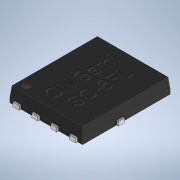
# Autodesk Inventor part: SO-8FL
Saved by Autodesk Inventor 2020.1 (Build 241239000, 239)
## iProperties
Created: 2020-03-12
Part Number: SO-8FL
Material: Generic
Document SubType Name: Modeling
Designer: yusaku
Density: 1 g/cm^3
Appearance: Default
Author: yusaku
Autodesk Inventor part; units mm, degrees
ref_plane "YZ Plane" through (0, 0, 0) normal (1, 0, 0) x (0, 1, 0)
ref_plane "XZ Plane" through (0, 0, 0) normal (0, 1, 0) x (-1, 0, 0)
ref_plane "Work Plane1" through (0, 0, 1) normal (0, 0, 1) x (1, 0, 0)
sketch "Sketch1" plane through (0, 0, 1) normal (0, 0, 1) x (1, 0, 0)
  line L0 (-2.45, 2.95) -> (2.45, 2.95)
  line L1 (2.45, 2.95) -> (2.45, -2.95)
  line L2 (2.45, -2.95) -> (-2.45, -2.95)
  line L3 (-2.45, -2.95) -> (-2.45, 2.95)
  point P0 (0, 0)
  point P1 (2.45, 0)
  point P2 (0, 2.95)
  dimension "d2" = 4.9
  dimension "d3" = 5.9
  constraints: 8 end point, 2 midpoint, 2 parallel, 1 horizontal, 1 horizontal alignment, 1 perpendicular, 1 vertical alignment
  measures "d2" distance of L0.start L0.end
  measures "d3" distance of L0.end L1.end
extrude "Extrusion1" add sketch "Sketch1" against normal blind 0.99
sketch "Sketch2" plane through (0, 0, 0) normal (0, 0, 1) x (1, 0, 0)
  line L0 (2.11, -2.5) -> (1.7, -2.5)
  line L1 (1.7, -2.5) -> (1.7, -3.075)
  line L2 (1.7, -3.075) -> (2.11, -3.075)
  line L3 (2.11, -3.075) -> (2.11, -2.5)
  line L4 (0.84, -2.5) -> (0.43, -2.5)
  line L5 (0.43, -2.5) -> (0.43, -3.075)
  line L6 (0.43, -3.075) -> (0.84, -3.075)
  line L7 (0.84, -3.075) -> (0.84, -2.5)
  line L8 (-0.43, -2.5) -> (-0.84, -2.5)
  line L9 (-0.84, -2.5) -> (-0.84, -3.075)
  line L10 (-0.84, -3.075) -> (-0.43, -3.075)
  line L11 (-0.43, -3.075) -> (-0.43, -2.5)
  line L12 (-1.7, -2.5) -> (-2.11, -2.5)
  line L13 (-2.11, -2.5) -> (-2.11, -3.075)
  line L14 (-2.11, -3.075) -> (-1.7, -3.075)
  line L15 (-1.7, -3.075) -> (-1.7, -2.5)
  line L16 (2.11, 3.075) -> (2.11, 2.075)
  line L17 (2.11, 2.075) -> (2, 2.075)
  line L18 (2, 2.075) -> (2, -0.245)
  line L19 (2, -0.245) -> (2.575, -0.245)
  line L20 (2.575, -0.245) -> (2.575, -0.655)
  line L21 (2.575, -0.655) -> (2, -0.655)
  line L22 (2, -0.655) -> (2, -1.15)
  line L23 (2, -1.15) -> (-2, -1.15)
  line L24 (-2, -1.15) -> (-2, -0.655)
  line L25 (-2, -0.655) -> (-2.575, -0.655)
  line L26 (-2.575, -0.655) -> (-2.575, -0.245)
  line L27 (-2.575, -0.245) -> (-2, -0.245)
  line L28 (-2, -0.245) -> (-2, 2.075)
  line L29 (-2.11, 2.075) -> (-2, 2.075)
  line L30 (-2.11, 2.075) -> (-2.11, 3.075)
  line L31 (2.11, 3.075) -> (1.7, 3.075)
  line L32 (1.7, 3.075) -> (1.7, 2.5)
  line L33 (1.7, 2.5) -> (-1.7, 2.5)
  line L34 (-1.7, 2.5) -> (-1.7, 3.075)
  line L35 (-1.7, 3.075) -> (-2.11, 3.075)
  line L36 (-0.635, -2.5) -> (-0.635, -3.075) construction
  line L37 (-1.905, -2.5) -> (-1.905, -3.075) construction
  line L38 (0.635, -2.5) -> (0.635, -3.075) construction
  line L39 (1.905, -2.5) -> (1.905, -3.075) construction
  line L40 (-2.45, 2.95) -> (2.45, 2.95) construction
  line L41 (0, 2.95) -> (0, -2.95) construction
  line L42 (2.45, -2.95) -> (-2.45, -2.95) construction
  line L43 (2.575, -0.45) -> (-2.575, -0.45) construction
  line L44 (-2.11, 2.075) -> (-2.11, -2.5) construction
  point P0 (0, 0)
  point P1 (0, -1.15)
  point P2 (0, 2.5)
  dimension "d6" = 0.635
  dimension "d7" = 1.27
  dimension "d10" = 1.27
  dimension "d11" = 1.35
  dimension "d12" = 0.575
  dimension "d13" = 6.15
  dimension "d14" = 5.15
  dimension "d15" = 0.125
  dimension "d16" = 3.4
  dimension "d17" = 4
  dimension "d18" = 0.41
  dimension "d19" = 0.575
  dimension "d20" = 1
  constraints: 86 end point, 19 point on line, 17 perpendicular, 14 midpoint, 8 parallel, 7 equal length, 5 horizontal, 3 vertical, 1 other
  measures "d6" distance from line of L36 point (0, 0)
  measures "d7" distance between parallel lines of L38 L36
  measures "d10" distance between parallel lines of L38 L39
  measures "d11" distance between parallel lines of L12 L23
  measures "d12" distance of L12.end L13.end
  measures "d13" distance between parallel lines of L2 L31
  measures "d14" distance between parallel lines of L26 L20
  measures "d15" distance between parallel lines of L40 L35
  measures "d16" distance between parallel lines of L40 L43
  measures "d17" distance between parallel lines of L18 L28
  measures "d18" distance of L13.end L14.end
  measures "d19" distance between parallel lines of L33 L31
  measures "d20" distance of L29.start L30.end
extrude "Extrusion2" add sketch "Sketch2" along normal blind 0.28
chamfer "Chamfer1" distance 0.0757 angle 84 4 edges at (0, 2.95, 1) (2.45, 0, 1) (0, -2.95, 1) (-2.45, 0, 1) measured on face at (0, -2.45, 1) measured on face at (1.95, 0, 1) measured on face at (0, 2.45, 1) measured on face at (-1.95, 0, 1)
sketch "Sketch3" plane through (0, 0, 1) normal (0, 0, 1) x (1, 0, 0)
  circle A0 centre (-1.8743, -2.3743) radius 0.25
  line L0 (2.3743, -2.8743) -> (-2.3743, -2.8743) projected
  line L1 (-2.3743, -2.8743) -> (-2.3743, 2.8743) projected
  line L2 (-0.981, -2.2668) -> (-0.981, 2.2668) construction
  line L3 (-0.981, 2.2668) -> (0.981, 2.2668) construction
  line L4 (0.981, 2.2668) -> (0.981, -2.2668) construction
  line L5 (0.981, -2.2668) -> (-0.981, -2.2668) construction
  spline S0 degree 2 poles (-0.5566, -2.2125) (-0.756, -2.2125) (-0.981, -1.9985) (-0.981, -1.8296) knots 0 0 0 1 2 2 2
  spline S1 degree 2 poles (-0.981, -1.8296) (-0.981, -1.7186) (-0.8749, -1.5405) (-0.6859, -1.4473) (-0.5657, -1.4473) knots 0 0 0 1 2 3 3 3
  spline S2 degree 2 poles (-0.5657, -1.4473) (-0.4444, -1.4473) (-0.2523, -1.5454) (-0.1535, -1.7259) (-0.1535, -1.8296) knots 0 0 0 1 2 3 3 3
  spline S3 degree 2 poles (-0.1535, -1.8296) (-0.1535, -1.943) (-0.2627, -2.121) (-0.4511, -2.2125) (-0.5566, -2.2125) knots 0 0 0 1 2 3 3 3
  spline S4 degree 2 poles (-0.5554, -2.1034) (-0.4109, -2.1034) (-0.2444, -1.9479) (-0.2444, -1.8302) knots 0 0 0 1 2 2 2
  spline S5 degree 2 poles (-0.2444, -1.8302) (-0.2444, -1.7107) (-0.4121, -1.5564) (-0.567, -1.5564) knots 0 0 0 1 2 2 2
  spline S6 degree 2 poles (-0.567, -1.5564) (-0.6645, -1.5564) (-0.8103, -1.6223) (-0.8901, -1.7497) (-0.8901, -1.829) knots 0 0 0 1 2 3 3 3
  spline S7 degree 2 poles (-0.8901, -1.829) (-0.8901, -1.9412) (-0.7359, -2.1034) (-0.5554, -2.1034) knots 0 0 0 1 2 2 2
  line L6 (-0.167, -1.3119) -> (-0.967, -1.3119)
  line L7 (-0.967, -1.3119) -> (-0.967, -1.2034)
  line L8 (-0.967, -1.2034) -> (-0.3389, -0.7826)
  line L9 (-0.3389, -0.7826) -> (-0.967, -0.7826)
  line L10 (-0.967, -0.7826) -> (-0.967, -0.6814)
  line L11 (-0.967, -0.6814) -> (-0.167, -0.6814)
  line L12 (-0.167, -0.6814) -> (-0.167, -0.7899)
  line L13 (-0.167, -0.7899) -> (-0.795, -1.2107)
  line L14 (-0.795, -1.2107) -> (-0.167, -1.2107)
  line L15 (-0.167, -1.2107) -> (-0.167, -1.3119)
  line L16 (-0.4243, -0.2296) -> (-0.4328, -0.1296)
  spline S8 degree 2 poles (-0.4328, -0.1296) (-0.3724, -0.1223) (-0.2956, -0.0704) (-0.2481, 0.0387) (-0.2481, 0.107) knots 0 0 0 1 2 3 3 3
  spline S9 degree 2 poles (-0.2481, 0.107) (-0.2481, 0.1674) (-0.284, 0.2607) (-0.3468, 0.3058) (-0.384, 0.3058) knots 0 0 0 1 2 3 3 3
  spline S10 degree 2 poles (-0.384, 0.3058) (-0.4218, 0.3058) (-0.4779, 0.2625) (-0.4968, 0.2119) knots 0 0 0 1 2 2 2
  spline S11 degree 2 poles (-0.4968, 0.2119) (-0.5096, 0.1796) (-0.5627, -0.0418) (-0.5865, -0.0863) knots 0 0 0 1 2 2 2
  spline S12 degree 2 poles (-0.5865, -0.0863) (-0.6164, -0.1436) (-0.7054, -0.1997) (-0.7603, -0.1997) knots 0 0 0 1 2 2 2
  spline S13 degree 2 poles (-0.7603, -0.1997) (-0.8212, -0.1997) (-0.9261, -0.1308) (-0.981, 0.0015) (-0.981, 0.0826) knots 0 0 0 1 2 3 3 3
  spline S14 degree 2 poles (-0.981, 0.0826) (-0.981, 0.1716) (-0.9237, 0.3076) (-0.8121, 0.3814) (-0.742, 0.3838) knots 0 0 0 1 2 3 3 3
  line L17 (-0.742, 0.3838) -> (-0.734, 0.2826)
  spline S15 degree 2 poles (-0.734, 0.2826) (-0.8103, 0.2747) (-0.8877, 0.1796) (-0.8877, 0.0869) knots 0 0 0 1 2 2 2
  spline S16 degree 2 poles (-0.8877, 0.0869) (-0.8877, -0.0095) (-0.817, -0.0979) (-0.7676, -0.0979) knots 0 0 0 1 2 2 2
  spline S17 degree 2 poles (-0.7676, -0.0979) (-0.7243, -0.0979) (-0.6962, -0.0668) knots 0 0 0 1 1 1
  spline S18 degree 2 poles (-0.6962, -0.0668) (-0.6688, -0.0357) (-0.6103, 0.2235) (-0.5883, 0.2716) knots 0 0 0 1 2 2 2
  spline S19 degree 2 poles (-0.5883, 0.2716) (-0.556, 0.3412) (-0.4572, 0.4076) (-0.3932, 0.4076) knots 0 0 0 1 2 2 2
  spline S20 degree 2 poles (-0.3932, 0.4076) (-0.3292, 0.4076) (-0.2164, 0.3345) (-0.1535, 0.1973) (-0.1535, 0.1119) knots 0 0 0 1 2 3 3 3
  spline S21 degree 2 poles (-0.1535, 0.1119) (-0.1535, 0.0027) (-0.217, -0.1436) (-0.3438, -0.2271) (-0.4243, -0.2296) knots 0 0 0 1 2 3 3 3
  line L18 (-0.3542, 0.9363) -> (-0.3414, 1.0381)
  spline S22 degree 2 poles (-0.3414, 1.0381) (-0.2523, 1.0137) (-0.1542, 0.8838) (-0.1542, 0.7832) knots 0 0 0 1 2 2 2
  spline S23 degree 2 poles (-0.1542, 0.7832) (-0.1542, 0.6558) (-0.3109, 0.507) (-0.4517, 0.507) knots 0 0 0 1 2 2 2
  spline S24 degree 2 poles (-0.4517, 0.507) (-0.5981, 0.507) (-0.7596, 0.6576) (-0.7596, 0.7777) knots 0 0 0 1 2 2 2
  spline S25 degree 2 poles (-0.7596, 0.7777) (-0.7596, 0.8936) (-0.6011, 1.0412) (-0.4578, 1.0412) knots 0 0 0 1 2 2 2
  spline S26 degree 2 poles (-0.4578, 1.0412) (-0.4493, 1.0412) (-0.4316, 1.0405) knots 0 0 0 1 1 1
  line L19 (-0.4316, 1.0405) -> (-0.4316, 0.6082)
  spline S27 degree 2 poles (-0.4316, 0.6082) (-0.3359, 0.6137) (-0.2346, 0.7107) (-0.2346, 0.7832) knots 0 0 0 1 2 2 2
  spline S28 degree 2 poles (-0.2346, 0.7832) (-0.2346, 0.8375) (-0.292, 0.9137) (-0.3542, 0.9363) knots 0 0 0 1 2 2 2
  line L20 (-0.5121, 0.6137) -> (-0.5121, 0.9375)
  spline S29 degree 2 poles (-0.5121, 0.9375) (-0.5853, 0.9308) (-0.6224, 0.9003) knots 0 0 0 1 1 1
  spline S30 degree 2 poles (-0.6224, 0.9003) (-0.6792, 0.8534) (-0.6792, 0.7784) knots 0 0 0 1 1 1
  spline S31 degree 2 poles (-0.6792, 0.7784) (-0.6792, 0.7107) (-0.5883, 0.6186) (-0.5121, 0.6137) knots 0 0 0 1 2 2 2
  line L21 (-0.167, 1.1613) -> (-0.7468, 1.1613)
  line L22 (-0.7468, 1.1613) -> (-0.7468, 1.2491)
  line L23 (-0.7468, 1.2491) -> (-0.6651, 1.2491)
  spline S32 degree 2 poles (-0.6651, 1.2491) (-0.7078, 1.2765) (-0.7596, 1.3668) (-0.7596, 1.4247) knots 0 0 0 1 2 2 2
  spline S33 degree 2 poles (-0.7596, 1.4247) (-0.7596, 1.4893) (-0.706, 1.5716) (-0.6578, 1.5887) knots 0 0 0 1 2 2 2
  spline S34 degree 2 poles (-0.6578, 1.5887) (-0.7596, 1.6576) (-0.7596, 1.768) knots 0 0 0 1 1 1
  spline S35 degree 2 poles (-0.7596, 1.768) (-0.7596, 1.854) (-0.6639, 1.9473) (-0.5645, 1.9473) knots 0 0 0 1 2 2 2
  line L24 (-0.5645, 1.9473) -> (-0.167, 1.9473)
  line L25 (-0.167, 1.9473) -> (-0.167, 1.8491)
  line L26 (-0.167, 1.8491) -> (-0.5322, 1.8491)
  spline S36 degree 2 poles (-0.5322, 1.8491) (-0.5907, 1.8491) (-0.6426, 1.8296) (-0.6743, 1.7796) (-0.6743, 1.746) knots 0 0 0 1 2 3 3 3
  spline S37 degree 2 poles (-0.6743, 1.746) (-0.6743, 1.6845) (-0.5932, 1.604) (-0.5035, 1.604) knots 0 0 0 1 2 2 2
  line L27 (-0.5035, 1.604) -> (-0.167, 1.604)
  line L28 (-0.167, 1.604) -> (-0.167, 1.5058)
  line L29 (-0.167, 1.5058) -> (-0.5432, 1.5058)
  spline S38 degree 2 poles (-0.5432, 1.5058) (-0.609, 1.5058) (-0.6743, 1.4576) (-0.6743, 1.4027) knots 0 0 0 1 2 2 2
  spline S39 degree 2 poles (-0.6743, 1.4027) (-0.6743, 1.3613) (-0.6304, 1.2912) (-0.5468, 1.2595) (-0.4676, 1.2595) knots 0 0 0 1 2 3 3 3
  line L30 (-0.4676, 1.2595) -> (-0.167, 1.2595)
  line L31 (-0.167, 1.2595) -> (-0.167, 1.1613)
  line L32 (-0.167, 2.093) -> (-0.7468, 2.093)
  line L33 (-0.7468, 2.093) -> (-0.7468, 2.1912)
  line L34 (-0.7468, 2.1912) -> (-0.167, 2.1912)
  line L35 (-0.167, 2.1912) -> (-0.167, 2.093)
  line L36 (-0.8542, 2.093) -> (-0.967, 2.093)
  line L37 (-0.967, 2.093) -> (-0.967, 2.1912)
  line L38 (-0.967, 2.1912) -> (-0.8542, 2.1912)
  line L39 (-0.8542, 2.1912) -> (-0.8542, 2.093)
  line L40 (0.8347, -1.9064) -> (0.8261, -1.8064)
  spline S40 degree 2 poles (0.8261, -1.8064) (0.8865, -1.7991) (0.9633, -1.7473) (1.0109, -1.6381) (1.0109, -1.5698) knots 0 0 0 1 2 3 3 3
  spline S41 degree 2 poles (1.0109, -1.5698) (1.0109, -1.5095) (0.9749, -1.4162) (0.9121, -1.371) (0.8749, -1.371) knots 0 0 0 1 2 3 3 3
  spline S42 degree 2 poles (0.8749, -1.371) (0.8371, -1.371) (0.781, -1.4143) (0.7621, -1.4649) knots 0 0 0 1 2 2 2
  spline S43 degree 2 poles (0.7621, -1.4649) (0.7493, -1.4973) (0.6963, -1.7186) (0.6725, -1.7631) knots 0 0 0 1 2 2 2
  spline S44 degree 2 poles (0.6725, -1.7631) (0.6426, -1.8204) (0.5536, -1.8765) (0.4987, -1.8765) knots 0 0 0 1 2 2 2
  spline S45 degree 2 poles (0.4987, -1.8765) (0.4377, -1.8765) (0.3329, -1.8076) (0.278, -1.6753) (0.278, -1.5942) knots 0 0 0 1 2 3 3 3
  spline S46 degree 2 poles (0.278, -1.5942) (0.278, -1.5052) (0.3353, -1.3692) (0.4469, -1.2954) (0.517, -1.293) knots 0 0 0 1 2 3 3 3
  line L41 (0.517, -1.293) -> (0.5249, -1.3942)
  spline S47 degree 2 poles (0.5249, -1.3942) (0.4487, -1.4021) (0.3713, -1.4973) (0.3713, -1.5899) knots 0 0 0 1 2 2 2
  spline S48 degree 2 poles (0.3713, -1.5899) (0.3713, -1.6863) (0.442, -1.7747) (0.4914, -1.7747) knots 0 0 0 1 2 2 2
  spline S49 degree 2 poles (0.4914, -1.7747) (0.5347, -1.7747) (0.5627, -1.7436) knots 0 0 0 1 1 1
  spline S50 degree 2 poles (0.5627, -1.7436) (0.5902, -1.7125) (0.6487, -1.4534) (0.6707, -1.4052) knots 0 0 0 1 2 2 2
  spline S51 degree 2 poles (0.6707, -1.4052) (0.703, -1.3357) (0.8018, -1.2692) (0.8658, -1.2692) knots 0 0 0 1 2 2 2
  spline S52 degree 2 poles (0.8658, -1.2692) (0.9298, -1.2692) (1.0426, -1.3424) (1.1054, -1.4796) (1.1054, -1.5649) knots 0 0 0 1 2 3 3 3
  spline S53 degree 2 poles (1.1054, -1.5649) (1.1054, -1.6741) (1.042, -1.8204) (0.9152, -1.904) (0.8347, -1.9064) knots 0 0 0 1 2 3 3 3
  spline S54 degree 2 poles (0.7024, -1.1564) (0.503, -1.1564) (0.278, -0.9424) (0.278, -0.7735) knots 0 0 0 1 2 2 2
  spline S55 degree 2 poles (0.278, -0.7735) (0.278, -0.6625) (0.3841, -0.4845) (0.5731, -0.3912) (0.6932, -0.3912) knots 0 0 0 1 2 3 3 3
  spline S56 degree 2 poles (0.6932, -0.3912) (0.8146, -0.3912) (1.0066, -0.4893) (1.1054, -0.6698) (1.1054, -0.7735) knots 0 0 0 1 2 3 3 3
  spline S57 degree 2 poles (1.1054, -0.7735) (1.1054, -0.8869) (0.9963, -1.0649) (0.8079, -1.1564) (0.7024, -1.1564) knots 0 0 0 1 2 3 3 3
  spline S58 degree 2 poles (0.7036, -1.0473) (0.8481, -1.0473) (1.0146, -0.8918) (1.0146, -0.7741) knots 0 0 0 1 2 2 2
  spline S59 degree 2 poles (1.0146, -0.7741) (1.0146, -0.6546) (0.8469, -0.5003) (0.692, -0.5003) knots 0 0 0 1 2 2 2
  spline S60 degree 2 poles (0.692, -0.5003) (0.5944, -0.5003) (0.4487, -0.5662) (0.3688, -0.6936) (0.3688, -0.7729) knots 0 0 0 1 2 3 3 3
  spline S61 degree 2 poles (0.3688, -0.7729) (0.3688, -0.8851) (0.5231, -1.0473) (0.7036, -1.0473) knots 0 0 0 1 2 2 2
  line L42 (0.8518, -0.3064) -> (0.753, -0.3064)
  line L43 (0.753, -0.3064) -> (0.753, -0.004)
  line L44 (0.753, -0.004) -> (0.8518, -0.004)
  line L45 (0.8518, -0.004) -> (0.8518, -0.3064)
  spline S62 degree 2 poles (0.6579, 0.229) (0.6353, 0.1674) (0.5524, 0.1082) (0.4951, 0.1082) knots 0 0 0 1 2 2 2
  spline S63 degree 2 poles (0.4951, 0.1082) (0.4079, 0.1082) (0.289, 0.2338) (0.289, 0.3375) knots 0 0 0 1 2 2 2
  spline S64 degree 2 poles (0.289, 0.3375) (0.289, 0.4424) (0.4103, 0.5698) (0.4975, 0.5698) knots 0 0 0 1 2 2 2
  spline S65 degree 2 poles (0.4975, 0.5698) (0.553, 0.5698) (0.6353, 0.5113) (0.6579, 0.4515) knots 0 0 0 1 2 2 2
  spline S66 degree 2 poles (0.6579, 0.4515) (0.6816, 0.5259) (0.789, 0.6027) (0.8633, 0.6027) knots 0 0 0 1 2 2 2
  spline S67 degree 2 poles (0.8633, 0.6027) (0.9658, 0.6027) (1.1054, 0.4576) (1.1054, 0.3393) knots 0 0 0 1 2 2 2
  spline S68 degree 2 poles (1.1054, 0.3393) (1.1054, 0.221) (0.9652, 0.0759) (0.8603, 0.0759) knots 0 0 0 1 2 2 2
  spline S69 degree 2 poles (0.8603, 0.0759) (0.7822, 0.0759) (0.6768, 0.1552) (0.6579, 0.229) knots 0 0 0 1 2 2 2
  spline S70 degree 2 poles (0.8609, 0.1771) (0.903, 0.1771) (0.9816, 0.2168) (1.0249, 0.2948) (1.0249, 0.3399) knots 0 0 0 1 2 3 3 3
  spline S71 degree 2 poles (1.0249, 0.3399) (1.0249, 0.4107) (0.9341, 0.5015) (0.8646, 0.5015) knots 0 0 0 1 2 2 2
  spline S72 degree 2 poles (0.8646, 0.5015) (0.7932, 0.5015) (0.7005, 0.4076) (0.7005, 0.3369) knots 0 0 0 1 2 2 2
  spline S73 degree 2 poles (0.7005, 0.3369) (0.7005, 0.2674) (0.792, 0.1771) (0.8609, 0.1771) knots 0 0 0 1 2 2 2
  spline S74 degree 2 poles (0.4914, 0.2095) (0.5481, 0.2095) (0.6201, 0.282) (0.6201, 0.3399) knots 0 0 0 1 2 2 2
  spline S75 degree 2 poles (0.6201, 0.3399) (0.6201, 0.3966) (0.5487, 0.4686) (0.4969, 0.4686) knots 0 0 0 1 2 2 2
  spline S76 degree 2 poles (0.4969, 0.4686) (0.4432, 0.4686) (0.3694, 0.3948) (0.3694, 0.3393) knots 0 0 0 1 2 2 2
  spline S77 degree 2 poles (0.3694, 0.3393) (0.3694, 0.2826) (0.4414, 0.2095) (0.4914, 0.2095) knots 0 0 0 1 2 2 2
  line L46 (1.092, 0.7436) -> (0.292, 0.7436)
  line L47 (0.292, 0.7436) -> (0.292, 1.2838)
  line L48 (0.292, 1.2838) -> (0.3865, 1.2838)
  line L49 (0.3865, 1.2838) -> (0.3865, 0.8497)
  line L50 (0.3865, 0.8497) -> (0.6341, 0.8497)
  line L51 (0.6341, 0.8497) -> (0.6341, 1.2253)
  line L52 (0.6341, 1.2253) -> (0.7286, 1.2253)
  line L53 (0.7286, 1.2253) -> (0.7286, 0.8497)
  line L54 (0.7286, 0.8497) -> (1.092, 0.8497)
  line L55 (1.092, 0.8497) -> (1.092, 0.7436)
  line L56 (1.092, 1.4168) -> (0.292, 1.4168)
  line L57 (0.292, 1.4168) -> (0.292, 1.5229)
  line L58 (0.292, 1.5229) -> (0.9975, 1.5229)
  line L59 (0.9975, 1.5229) -> (0.9975, 1.9168)
  line L60 (0.9975, 1.9168) -> (1.092, 1.9168)
  line L61 (1.092, 1.9168) -> (1.092, 1.4168)
  point P0 (0, 0)
  point P1 (0.981, 0)
  point P2 (0, 2.2668)
  dimension "d26" = 0.5
  dimension "d27" = 0.5
  dimension "d28" = 0.5
  constraints: 2 midpoint, 1 centre point, 1 horizontal alignment, 1 vertical alignment, 2 other
  measures "d26" diameter of A0
  measures "d27" distance from line of L0 A0.centre
  measures "d28" distance from line of L1 A0.centre
extrude "Extrusion3" cut sketch "Sketch3" against normal blind 0.1
equation "\"d2\" = dim_D1"
equation "\"d3\" = dim_E1"
equation "\"d4\" = dim_A - dim_A1"
equation "\"d6\" = 0.5 * dim_e"
equation "\"d7\" = dim_e"
equation "\"d10\" = dim_e"
equation "\"d11\" = dim_K"
equation "\"d12\" = dim_L"
equation "\"d13\" = dim_E"
equation "\"d14\" = dim_D"
equation "\"d15\" = dim_L1"
equation "\"d16\" = dim_M"
equation "\"d17\" = dim_D2"
equation "\"d18\" = dim_b"
equation "\"d19\" = dim_G"
equation "\"d21\" = dim_c"
equation "\"dim_A\" = 1"
equation "\"dim_A1\" = 0.01"
equation "\"dim_b\" = 0.41"
equation "\"dim_c\" = 0.28"
equation "\"dim_D\" = 5.15"
equation "\"dim_D1\" = 4.9"
equation "\"dim_D2\" = 4"
equation "\"dim_E\" = 6.15"
equation "\"dim_E1\" = 5.9"
equation "\"dim_E2\" = 3.65"
equation "\"dim_e\" = 1.27"
equation "\"dim_G\" = 0.575"
equation "\"dim_K\" = 1.35"
equation "\"dim_L\" = 0.575"
equation "\"dim_L1\" = 0.125"
equation "\"dim_M\" = 3.4"
equation "\"dim_theta\" = 6deg"
equation "\"d1\" = dim_A"
body "Solid1"
